Autodesk Inventor part; units mm, degrees
(part 3 of 3)
  point P86 (13.5104, 46.8405)
  point P87 (13.2211, 47.2236)
  point P88 (11.1615, 47.7468)
  point P89 (10.7263, 47.5553)
  point P90 (10.5426, 47.5964)
  point P91 (10.2298, 47.9606)
  point P92 (7.7191, 48.135)
  point P93 (7.5332, 48.1644)
  point P94 (7.1982, 48.5083)
  point P95 (5.0892, 48.7692)
  point P96 (4.6815, 48.5247)
  point P97 (4.4941, 48.5424)
  point P98 (4.1381, 48.8646)
  point P99 (2.0169, 48.9926)
  point P100 (1.6254, 48.7229)
  point P101 (1.4372, 48.7288)
  point P102 (1.0617, 49.028)
  point P103 (-1.0633, 49.0225)
  point P104 (-1.4372, 48.7288)
  point P105 (-1.6254, 48.7229)
  point P106 (-2.0189, 48.9979)
  point P107 (-2.8249, 50.9218)
  point P108 (-4.1394, 48.859)
  point P109 (-4.4941, 48.5424)
  point P110 (-4.6815, 48.5247)
  point P111 (-5.0915, 48.7745)
  point P112 (-6.0168, 50.6439)
  point P113 (-7.5332, 48.1644)
  point P114 (-7.7191, 48.135)
  point P115 (-8.144, 48.3585)
  point P116 (-9.1848, 50.1662)
  point P117 (-10.5426, 47.5964)
  point P118 (-10.7263, 47.5553)
  point P119 (-11.1644, 47.7517)
  point P120 (-12.3167, 49.4905)
  point P121 (-13.5104, 46.8405)
  point P122 (-13.6912, 46.788)
  point P123 (-14.1407, 46.9565)
  point P124 (-15.3999, 48.6194)
  point P125 (-16.1601, 46.2946)
  point P126 (-16.4249, 45.8997)
  point P127 (-16.602, 45.836)
  point P128 (-17.0612, 45.9759)
  point P129 (-18.4224, 47.5565)
  point P130 (-19.2745, 44.7778)
  point P131 (-19.4473, 44.7031)
  point P132 (-19.9144, 44.8139)
  point P133 (-21.3721, 46.3059)
  point P134 (-21.8349, 43.9042)
  point P135 (-22.0481, 43.4792)
  point P136 (-22.2159, 43.3938)
  point P137 (-24.2375, 44.8726)
  point P138 (-24.7347, 42.009)
  point P139 (-24.8967, 41.9132)
  point P140 (-25.3741, 41.9646)
  point P141 (-27.0072, 43.2622)
  point P142 (-27.1654, 40.8213)
  point P143 (-27.3237, 40.373)
  point P144 (-27.4794, 40.2672)
  point P145 (-27.959, 40.2885)
  point P146 (-29.6704, 41.481)
  point P147 (-29.6769, 39.0404)
  point P148 (-29.8048, 38.5777)
  point P149 (-29.9535, 38.4623)
  point P150 (-30.4336, 38.4535)
  point P151 (-32.0674, 37.0947)
  point P152 (-32.1683, 36.6301)
  point P153 (-32.3095, 36.5056)
  point P154 (-32.788, 36.4667)
  point P155 (-34.6354, 37.4352)
  point P156 (-34.4048, 34.5379)
  point P157 (-34.5379, 34.4048)
  point P158 (-35.0131, 34.3359)
  point P159 (-36.9176, 35.1866)
  point P160 (-36.5056, 32.3095)
  point P161 (-36.6301, 32.1683)
  point P162 (-37.1, 32.0697)
  point P163 (-39.0542, 32.7991)
  point P164 (-38.4623, 29.9535)
  point P165 (-38.5777, 29.8048)
  point P166 (-39.0404, 29.6769)
  point P167 (-41.0366, 30.2821)
  point P168 (-40.2851, 27.9545)
  point P169 (-40.2672, 27.4794)
  point P170 (-40.373, 27.3237)
  point P171 (-40.8268, 27.1669)
  point P172 (-42.857, 27.6457)
  point P173 (-41.9132, 24.8967)
  point P174 (-42.009, 24.7347)
  point P175 (-42.4521, 24.5498)
  point P176 (-43.471, 22.685)
  point P177 (-43.3938, 22.2159)
  point P178 (-43.4792, 22.0481)
  point P179 (-43.9098, 21.8358)
  point P180 (-45.984, 22.0563)
  point P181 (-44.7031, 19.4473)
  point P182 (-44.7778, 19.2745)
  point P183 (-45.1942, 19.0356)
  point P184 (-47.2782, 19.1254)
  point P185 (-45.836, 16.602)
  point P186 (-45.8997, 16.4249)
  point P187 (-46.3003, 16.1602)
  point P188 (-48.3858, 16.119)
  point P189 (-46.788, 13.6912)
  point P190 (-46.8405, 13.5104)
  point P191 (-47.2236, 13.2211)
  point P192 (-47.7468, 11.1615)
  point P193 (-47.5553, 10.7263)
  point P194 (-47.5964, 10.5426)
  point P195 (-47.9606, 10.2298)
  point P196 (-50.0245, 9.9276)
  point P197 (-48.135, 7.7191)
  point P198 (-48.1644, 7.5332)
  point P199 (-48.5083, 7.1982)
  constraints: 800 point on circle, 400 centre point, 600 other
extrude "Extrusion1" add sketch "Sketch1" along normal blind 7
sketch "Sketch10" plane through (0, 0, 7) normal (0, 0, 1) x (1, 0, 0)
  arc A0 (8.9575, -3.1642) -> (9.3396, -1.7385) centre (0, 0) ccw
  arc A1 (9.7901, -1.4158) -> (9.3396, -1.7385) centre (9.7328, -1.8117) ccw
  line L0 (9.7901, -1.4158) -> (11.1918, -1.6185)
  spline S0 degree 3 poles (11.1918, -1.6185) (11.2745, -1.6242) (11.5228, -1.6292) (11.9415, -1.5322) knots 0 0 0 0 1 1 1 1
  line L1 (11.1918, -1.6185) -> (11.2745, -1.6242) construction
  line L2 (11.2745, -1.6242) -> (11.5228, -1.6292) construction
  line L3 (11.5228, -1.6292) -> (11.9415, -1.5322) construction
  spline S1 degree 3 poles (11.9415, -1.5322) (12.4367, -1.4162) (13.1438, -1.1571) (13.9903, -0.5909) knots 0 0 0 0 1 1 1 1
  line L4 (11.9415, -1.5322) -> (12.4367, -1.4162) construction
  line L5 (12.4367, -1.4162) -> (13.1438, -1.1571) construction
  line L6 (13.1438, -1.1571) -> (13.9903, -0.5909) construction
  arc A2 (13.9903, -0.5909) -> (13.9903, 0.5909) centre (0, 0) ccw
  spline S2 degree 3 poles (13.9903, 0.5909) (13.1438, 1.1571) (12.4367, 1.4162) (11.9415, 1.5322) knots 0 0 0 0 1 1 1 1
  line L7 (13.9903, 0.5909) -> (13.1438, 1.1571) construction
  line L8 (13.1438, 1.1571) -> (12.4367, 1.4162) construction
  line L9 (12.4367, 1.4162) -> (11.9415, 1.5322) construction
  spline S3 degree 3 poles (11.9415, 1.5322) (11.5228, 1.6292) (11.2745, 1.6242) (11.1918, 1.6185) knots 0 0 0 0 1 1 1 1
  line L10 (11.9415, 1.5322) -> (11.5228, 1.6292) construction
  line L11 (11.5228, 1.6292) -> (11.2745, 1.6242) construction
  line L12 (11.2745, 1.6242) -> (11.1918, 1.6185) construction
  line L13 (11.1918, 1.6185) -> (9.7901, 1.4158)
  arc A3 (9.3396, 1.7385) -> (9.7901, 1.4158) centre (9.7328, 1.8117) ccw
  arc A4 (9.3396, 1.7385) -> (8.9575, 3.1642) centre (0, 0) ccw
  arc A5 (9.1863, 3.6689) -> (8.9575, 3.1642) centre (9.3347, 3.2975) ccw
  line L14 (9.1863, 3.6689) -> (10.5016, 4.1942)
  spline S4 degree 3 poles (10.5016, 4.1942) (10.5761, 4.2307) (10.7937, 4.3505) (11.1078, 4.6438) knots 0 0 0 0 1 1 1 1
  line L15 (10.5016, 4.1942) -> (10.5761, 4.2307) construction
  line L16 (10.5761, 4.2307) -> (10.7937, 4.3505) construction
  line L17 (10.7937, 4.3505) -> (11.1078, 4.6438) construction
  spline S5 degree 3 poles (11.1078, 4.6438) (11.4787, 4.9919) (11.9614, 5.5698) (12.4114, 6.4834) knots 0 0 0 0 1 1 1 1
  line L18 (11.1078, 4.6438) -> (11.4787, 4.9919) construction
  line L19 (11.4787, 4.9919) -> (11.9614, 5.5698) construction
  line L20 (11.9614, 5.5698) -> (12.4114, 6.4834) construction
  arc A6 (12.4114, 6.4834) -> (11.8204, 7.5069) centre (0, 0) ccw
  spline S6 degree 3 poles (11.8204, 7.5069) (10.8043, 7.5739) (10.0624, 7.4449) (9.5755, 7.2977) knots 0 0 0 0 1 1 1 1
  line L21 (11.8204, 7.5069) -> (10.8043, 7.5739) construction
  line L22 (10.8043, 7.5739) -> (10.0624, 7.4449) construction
  line L23 (10.0624, 7.4449) -> (9.5755, 7.2977) construction
  spline S7 degree 3 poles (9.5755, 7.2977) (9.1645, 7.1723) (8.9519, 7.0438) (8.8831, 6.9975) knots 0 0 0 0 1 1 1 1
  line L24 (9.5755, 7.2977) -> (9.1645, 7.1723) construction
  line L25 (9.1645, 7.1723) -> (8.9519, 7.0438) construction
  line L26 (8.9519, 7.0438) -> (8.8831, 6.9975) construction
  line L27 (8.8831, 6.9975) -> (7.7706, 6.1211)
  arc A7 (7.2191, 6.1753) -> (7.7706, 6.1211) centre (7.523, 6.4354) ccw
  arc A8 (7.2191, 6.1753) -> (6.1753, 7.2191) centre (0, 0) ccw
  arc A9 (6.1211, 7.7706) -> (6.1753, 7.2191) centre (6.4354, 7.523) ccw
  line L28 (6.1211, 7.7706) -> (6.9975, 8.8831)
  spline S8 degree 3 poles (6.9975, 8.8831) (7.0438, 8.9519) (7.1723, 9.1645) (7.2977, 9.5755) knots 0 0 0 0 1 1 1 1
  line L29 (6.9975, 8.8831) -> (7.0438, 8.9519) construction
  line L30 (7.0438, 8.9519) -> (7.1723, 9.1645) construction
  line L31 (7.1723, 9.1645) -> (7.2977, 9.5755) construction
  spline S9 degree 3 poles (7.2977, 9.5755) (7.4449, 10.0624) (7.5739, 10.8043) (7.5069, 11.8204) knots 0 0 0 0 1 1 1 1
  line L32 (7.2977, 9.5755) -> (7.4449, 10.0624) construction
  line L33 (7.4449, 10.0624) -> (7.5739, 10.8043) construction
  line L34 (7.5739, 10.8043) -> (7.5069, 11.8204) construction
  arc A10 (7.5069, 11.8204) -> (6.4834, 12.4114) centre (0, 0) ccw
  spline S10 degree 3 poles (6.4834, 12.4114) (5.5698, 11.9614) (4.9919, 11.4787) (4.6438, 11.1078) knots 0 0 0 0 1 1 1 1
  line L35 (6.4834, 12.4114) -> (5.5698, 11.9614) construction
  line L36 (5.5698, 11.9614) -> (4.9919, 11.4787) construction
  line L37 (4.9919, 11.4787) -> (4.6438, 11.1078) construction
  spline S11 degree 3 poles (4.6438, 11.1078) (4.3505, 10.7937) (4.2307, 10.5761) (4.1942, 10.5016) knots 0 0 0 0 1 1 1 1
  line L38 (4.6438, 11.1078) -> (4.3505, 10.7937) construction
  line L39 (4.3505, 10.7937) -> (4.2307, 10.5761) construction
  line L40 (4.2307, 10.5761) -> (4.1942, 10.5016) construction
  line L41 (4.1942, 10.5016) -> (3.6689, 9.1863)
  arc A11 (3.1642, 8.9575) -> (3.6689, 9.1863) centre (3.2975, 9.3347) ccw
  arc A12 (3.1642, 8.9575) -> (1.7385, 9.3396) centre (0, 0) ccw
  arc A13 (1.4158, 9.7901) -> (1.7385, 9.3396) centre (1.8117, 9.7328) ccw
  line L42 (1.4158, 9.7901) -> (1.6185, 11.1918)
  spline S12 degree 3 poles (1.6185, 11.1918) (1.6242, 11.2745) (1.6292, 11.5228) (1.5322, 11.9415) knots 0 0 0 0 1 1 1 1
  line L43 (1.6185, 11.1918) -> (1.6242, 11.2745) construction
  line L44 (1.6242, 11.2745) -> (1.6292, 11.5228) construction
  line L45 (1.6292, 11.5228) -> (1.5322, 11.9415) construction
  spline S13 degree 3 poles (1.5322, 11.9415) (1.4162, 12.4367) (1.1571, 13.1438) (0.5909, 13.9903) knots 0 0 0 0 1 1 1 1
  line L46 (1.5322, 11.9415) -> (1.4162, 12.4367) construction
  line L47 (1.4162, 12.4367) -> (1.1571, 13.1438) construction
  line L48 (1.1571, 13.1438) -> (0.5909, 13.9903) construction
  arc A14 (0.5909, 13.9903) -> (-0.5909, 13.9903) centre (0, 0) ccw
  spline S14 degree 3 poles (-0.5909, 13.9903) (-1.1571, 13.1438) (-1.4162, 12.4367) (-1.5322, 11.9415) knots 0 0 0 0 1 1 1 1
  line L49 (-0.5909, 13.9903) -> (-1.1571, 13.1438) construction
  line L50 (-1.1571, 13.1438) -> (-1.4162, 12.4367) construction
  line L51 (-1.4162, 12.4367) -> (-1.5322, 11.9415) construction
  spline S15 degree 3 poles (-1.5322, 11.9415) (-1.6292, 11.5228) (-1.6242, 11.2745) (-1.6185, 11.1918) knots 0 0 0 0 1 1 1 1
  line L52 (-1.5322, 11.9415) -> (-1.6292, 11.5228) construction
  line L53 (-1.6292, 11.5228) -> (-1.6242, 11.2745) construction
  line L54 (-1.6242, 11.2745) -> (-1.6185, 11.1918) construction
  line L55 (-1.6185, 11.1918) -> (-1.4158, 9.7901)
  arc A15 (-1.7385, 9.3396) -> (-1.4158, 9.7901) centre (-1.8117, 9.7328) ccw
  arc A16 (-1.7385, 9.3396) -> (-3.1642, 8.9575) centre (0, 0) ccw
  arc A17 (-3.6689, 9.1863) -> (-3.1642, 8.9575) centre (-3.2975, 9.3347) ccw
  line L56 (-3.6689, 9.1863) -> (-4.1942, 10.5016)
  spline S16 degree 3 poles (-4.1942, 10.5016) (-4.2307, 10.5761) (-4.3505, 10.7937) (-4.6438, 11.1078) knots 0 0 0 0 1 1 1 1
  line L57 (-4.1942, 10.5016) -> (-4.2307, 10.5761) construction
  line L58 (-4.2307, 10.5761) -> (-4.3505, 10.7937) construction
  line L59 (-4.3505, 10.7937) -> (-4.6438, 11.1078) construction
  spline S17 degree 3 poles (-4.6438, 11.1078) (-4.9919, 11.4787) (-5.5698, 11.9614) (-6.4834, 12.4114) knots 0 0 0 0 1 1 1 1
  line L60 (-4.6438, 11.1078) -> (-4.9919, 11.4787) construction
  line L61 (-4.9919, 11.4787) -> (-5.5698, 11.9614) construction
  line L62 (-5.5698, 11.9614) -> (-6.4834, 12.4114) construction
  arc A18 (-6.4834, 12.4114) -> (-7.5069, 11.8204) centre (0, 0) ccw
  spline S18 degree 3 poles (-7.5069, 11.8204) (-7.5739, 10.8043) (-7.4449, 10.0624) (-7.2977, 9.5755) knots 0 0 0 0 1 1 1 1
  line L63 (-7.5069, 11.8204) -> (-7.5739, 10.8043) construction
  line L64 (-7.5739, 10.8043) -> (-7.4449, 10.0624) construction
  line L65 (-7.4449, 10.0624) -> (-7.2977, 9.5755) construction
  spline S19 degree 3 poles (-7.2977, 9.5755) (-7.1723, 9.1645) (-7.0438, 8.9519) (-6.9975, 8.8831) knots 0 0 0 0 1 1 1 1
  line L66 (-7.2977, 9.5755) -> (-7.1723, 9.1645) construction
  line L67 (-7.1723, 9.1645) -> (-7.0438, 8.9519) construction
  line L68 (-7.0438, 8.9519) -> (-6.9975, 8.8831) construction
  line L69 (-6.9975, 8.8831) -> (-6.1211, 7.7706)
  arc A19 (-6.1753, 7.2191) -> (-6.1211, 7.7706) centre (-6.4354, 7.523) ccw
  arc A20 (-6.1753, 7.2191) -> (-7.2191, 6.1753) centre (0, 0) ccw
  arc A21 (-7.7706, 6.1211) -> (-7.2191, 6.1753) centre (-7.523, 6.4354) ccw
  line L70 (-7.7706, 6.1211) -> (-8.8831, 6.9975)
  spline S20 degree 3 poles (-8.8831, 6.9975) (-8.9519, 7.0438) (-9.1645, 7.1723) (-9.5755, 7.2977) knots 0 0 0 0 1 1 1 1
  line L71 (-8.8831, 6.9975) -> (-8.9519, 7.0438) construction
  line L72 (-8.9519, 7.0438) -> (-9.1645, 7.1723) construction
  line L73 (-9.1645, 7.1723) -> (-9.5755, 7.2977) construction
  spline S21 degree 3 poles (-9.5755, 7.2977) (-10.0624, 7.4449) (-10.8043, 7.5739) (-11.8204, 7.5069) knots 0 0 0 0 1 1 1 1
  line L74 (-9.5755, 7.2977) -> (-10.0624, 7.4449) construction
  line L75 (-10.0624, 7.4449) -> (-10.8043, 7.5739) construction
  line L76 (-10.8043, 7.5739) -> (-11.8204, 7.5069) construction
  arc A22 (-11.8204, 7.5069) -> (-12.4114, 6.4834) centre (0, 0) ccw
  spline S22 degree 3 poles (-12.4114, 6.4834) (-11.9614, 5.5698) (-11.4787, 4.9919) (-11.1078, 4.6438) knots 0 0 0 0 1 1 1 1
  line L77 (-12.4114, 6.4834) -> (-11.9614, 5.5698) construction
  line L78 (-11.9614, 5.5698) -> (-11.4787, 4.9919) construction
  line L79 (-11.4787, 4.9919) -> (-11.1078, 4.6438) construction
  spline S23 degree 3 poles (-11.1078, 4.6438) (-10.7937, 4.3505) (-10.5761, 4.2307) (-10.5016, 4.1942) knots 0 0 0 0 1 1 1 1
  line L80 (-11.1078, 4.6438) -> (-10.7937, 4.3505) construction
  line L81 (-10.7937, 4.3505) -> (-10.5761, 4.2307) construction
  line L82 (-10.5761, 4.2307) -> (-10.5016, 4.1942) construction
  line L83 (-10.5016, 4.1942) -> (-9.1863, 3.6689)
  arc A23 (-8.9575, 3.1642) -> (-9.1863, 3.6689) centre (-9.3347, 3.2975) ccw
  arc A24 (-8.9575, 3.1642) -> (-9.3396, 1.7385) centre (0, 0) ccw
  arc A25 (-9.7901, 1.4158) -> (-9.3396, 1.7385) centre (-9.7328, 1.8117) ccw
  line L84 (-9.7901, 1.4158) -> (-11.1918, 1.6185)
  spline S24 degree 3 poles (-11.1918, 1.6185) (-11.2745, 1.6242) (-11.5228, 1.6292) (-11.9415, 1.5322) knots 0 0 0 0 1 1 1 1
  line L85 (-11.1918, 1.6185) -> (-11.2745, 1.6242) construction
  line L86 (-11.2745, 1.6242) -> (-11.5228, 1.6292) construction
  line L87 (-11.5228, 1.6292) -> (-11.9415, 1.5322) construction
  spline S25 degree 3 poles (-11.9415, 1.5322) (-12.4367, 1.4162) (-13.1438, 1.1571) (-13.9903, 0.5909) knots 0 0 0 0 1 1 1 1
  line L88 (-11.9415, 1.5322) -> (-12.4367, 1.4162) construction
  line L89 (-12.4367, 1.4162) -> (-13.1438, 1.1571) construction
  line L90 (-13.1438, 1.1571) -> (-13.9903, 0.5909) construction
  arc A26 (-13.9903, 0.5909) -> (-13.9903, -0.5909) centre (0, 0) ccw
  spline S26 degree 3 poles (-13.9903, -0.5909) (-13.1438, -1.1571) (-12.4367, -1.4162) (-11.9415, -1.5322) knots 0 0 0 0 1 1 1 1
  line L91 (-13.9903, -0.5909) -> (-13.1438, -1.1571) construction
  line L92 (-13.1438, -1.1571) -> (-12.4367, -1.4162) construction
  line L93 (-12.4367, -1.4162) -> (-11.9415, -1.5322) construction
  spline S27 degree 3 poles (-11.9415, -1.5322) (-11.5228, -1.6292) (-11.2745, -1.6242) (-11.1918, -1.6185) knots 0 0 0 0 1 1 1 1
  line L94 (-11.9415, -1.5322) -> (-11.5228, -1.6292) construction
  line L95 (-11.5228, -1.6292) -> (-11.2745, -1.6242) construction
  line L96 (-11.2745, -1.6242) -> (-11.1918, -1.6185) construction
  line L97 (-11.1918, -1.6185) -> (-9.7901, -1.4158)
  arc A27 (-9.3396, -1.7385) -> (-9.7901, -1.4158) centre (-9.7328, -1.8117) ccw
  arc A28 (-9.3396, -1.7385) -> (-8.9575, -3.1642) centre (0, 0) ccw
  arc A29 (-9.1863, -3.6689) -> (-8.9575, -3.1642) centre (-9.3347, -3.2975) ccw
  line L98 (-9.1863, -3.6689) -> (-10.5016, -4.1942)
  spline S28 degree 3 poles (-10.5016, -4.1942) (-10.5761, -4.2307) (-10.7937, -4.3505) (-11.1078, -4.6438) knots 0 0 0 0 1 1 1 1
  line L99 (-10.5016, -4.1942) -> (-10.5761, -4.2307) construction
  line L100 (-10.5761, -4.2307) -> (-10.7937, -4.3505) construction
  line L101 (-10.7937, -4.3505) -> (-11.1078, -4.6438) construction
  spline S29 degree 3 poles (-11.1078, -4.6438) (-11.4787, -4.9919) (-11.9614, -5.5698) (-12.4114, -6.4834) knots 0 0 0 0 1 1 1 1
  line L102 (-11.1078, -4.6438) -> (-11.4787, -4.9919) construction
  line L103 (-11.4787, -4.9919) -> (-11.9614, -5.5698) construction
  line L104 (-11.9614, -5.5698) -> (-12.4114, -6.4834) construction
  arc A30 (-12.4114, -6.4834) -> (-11.8204, -7.5069) centre (0, 0) ccw
  spline S30 degree 3 poles (-11.8204, -7.5069) (-10.8043, -7.5739) (-10.0624, -7.4449) (-9.5755, -7.2977) knots 0 0 0 0 1 1 1 1
  line L105 (-11.8204, -7.5069) -> (-10.8043, -7.5739) construction
  line L106 (-10.8043, -7.5739) -> (-10.0624, -7.4449) construction
  line L107 (-10.0624, -7.4449) -> (-9.5755, -7.2977) construction
  spline S31 degree 3 poles (-9.5755, -7.2977) (-9.1645, -7.1723) (-8.9519, -7.0438) (-8.8831, -6.9975) knots 0 0 0 0 1 1 1 1
  line L108 (-9.5755, -7.2977) -> (-9.1645, -7.1723) construction
  line L109 (-9.1645, -7.1723) -> (-8.9519, -7.0438) construction
  line L110 (-8.9519, -7.0438) -> (-8.8831, -6.9975) construction
  line L111 (-8.8831, -6.9975) -> (-7.7706, -6.1211)
  arc A31 (-7.2191, -6.1753) -> (-7.7706, -6.1211) centre (-7.523, -6.4354) ccw
  arc A32 (-7.2191, -6.1753) -> (-6.1753, -7.2191) centre (0, 0) ccw
  arc A33 (-6.1211, -7.7706) -> (-6.1753, -7.2191) centre (-6.4354, -7.523) ccw
  line L112 (-6.1211, -7.7706) -> (-6.9975, -8.8831)
  spline S32 degree 3 poles (-6.9975, -8.8831) (-7.0438, -8.9519) (-7.1723, -9.1645) (-7.2977, -9.5755) knots 0 0 0 0 1 1 1 1
  line L113 (-6.9975, -8.8831) -> (-7.0438, -8.9519) construction
  line L114 (-7.0438, -8.9519) -> (-7.1723, -9.1645) construction
  line L115 (-7.1723, -9.1645) -> (-7.2977, -9.5755) construction
  spline S33 degree 3 poles (-7.2977, -9.5755) (-7.4449, -10.0624) (-7.5739, -10.8043) (-7.5069, -11.8204) knots 0 0 0 0 1 1 1 1
  line L116 (-7.2977, -9.5755) -> (-7.4449, -10.0624) construction
  line L117 (-7.4449, -10.0624) -> (-7.5739, -10.8043) construction
  line L118 (-7.5739, -10.8043) -> (-7.5069, -11.8204) construction
  arc A34 (-7.5069, -11.8204) -> (-6.4834, -12.4114) centre (0, 0) ccw
  spline S34 degree 3 poles (-6.4834, -12.4114) (-5.5698, -11.9614) (-4.9919, -11.4787) (-4.6438, -11.1078) knots 0 0 0 0 1 1 1 1
  line L119 (-6.4834, -12.4114) -> (-5.5698, -11.9614) construction
  line L120 (-5.5698, -11.9614) -> (-4.9919, -11.4787) construction
  line L121 (-4.9919, -11.4787) -> (-4.6438, -11.1078) construction
  spline S35 degree 3 poles (-4.6438, -11.1078) (-4.3505, -10.7937) (-4.2307, -10.5761) (-4.1942, -10.5016) knots 0 0 0 0 1 1 1 1
  line L122 (-4.6438, -11.1078) -> (-4.3505, -10.7937) construction
  line L123 (-4.3505, -10.7937) -> (-4.2307, -10.5761) construction
  line L124 (-4.2307, -10.5761) -> (-4.1942, -10.5016) construction
  line L125 (-4.1942, -10.5016) -> (-3.6689, -9.1863)
  arc A35 (-3.1642, -8.9575) -> (-3.6689, -9.1863) centre (-3.2975, -9.3347) ccw
  arc A36 (-3.1642, -8.9575) -> (-1.7385, -9.3396) centre (0, 0) ccw
  arc A37 (-1.4158, -9.7901) -> (-1.7385, -9.3396) centre (-1.8117, -9.7328) ccw
  line L126 (-1.4158, -9.7901) -> (-1.6185, -11.1918)
  spline S36 degree 3 poles (-1.6185, -11.1918) (-1.6242, -11.2745) (-1.6292, -11.5228) (-1.5322, -11.9415) knots 0 0 0 0 1 1 1 1
  line L127 (-1.6185, -11.1918) -> (-1.6242, -11.2745) construction
  line L128 (-1.6242, -11.2745) -> (-1.6292, -11.5228) construction
  line L129 (-1.6292, -11.5228) -> (-1.5322, -11.9415) construction
  spline S37 degree 3 poles (-1.5322, -11.9415) (-1.4162, -12.4367) (-1.1571, -13.1438) (-0.5909, -13.9903) knots 0 0 0 0 1 1 1 1
  line L130 (-1.5322, -11.9415) -> (-1.4162, -12.4367) construction
  line L131 (-1.4162, -12.4367) -> (-1.1571, -13.1438) construction
  line L132 (-1.1571, -13.1438) -> (-0.5909, -13.9903) construction
  arc A38 (-0.5909, -13.9903) -> (0.5909, -13.9903) centre (0, 0) ccw
  spline S38 degree 3 poles (0.5909, -13.9903) (1.1571, -13.1438) (1.4162, -12.4367) (1.5322, -11.9415) knots 0 0 0 0 1 1 1 1
  line L133 (0.5909, -13.9903) -> (1.1571, -13.1438) construction
  line L134 (1.1571, -13.1438) -> (1.4162, -12.4367) construction
  line L135 (1.4162, -12.4367) -> (1.5322, -11.9415) construction
  spline S39 degree 3 poles (1.5322, -11.9415) (1.6292, -11.5228) (1.6242, -11.2745) (1.6185, -11.1918) knots 0 0 0 0 1 1 1 1
  line L136 (1.5322, -11.9415) -> (1.6292, -11.5228) construction
  line L137 (1.6292, -11.5228) -> (1.6242, -11.2745) construction
  line L138 (1.6242, -11.2745) -> (1.6185, -11.1918) construction
  line L139 (1.6185, -11.1918) -> (1.4158, -9.7901)
  arc A39 (1.7385, -9.3396) -> (1.4158, -9.7901) centre (1.8117, -9.7328) ccw
  arc A40 (1.7385, -9.3396) -> (3.1642, -8.9575) centre (0, 0) ccw
  arc A41 (3.6689, -9.1863) -> (3.1642, -8.9575) centre (3.2975, -9.3347) ccw
  line L140 (3.6689, -9.1863) -> (4.1942, -10.5016)
  spline S40 degree 3 poles (4.1942, -10.5016) (4.2307, -10.5761) (4.3505, -10.7937) (4.6438, -11.1078) knots 0 0 0 0 1 1 1 1
  line L141 (4.1942, -10.5016) -> (4.2307, -10.5761) construction
  line L142 (4.2307, -10.5761) -> (4.3505, -10.7937) construction
  line L143 (4.3505, -10.7937) -> (4.6438, -11.1078) construction
  spline S41 degree 3 poles (4.6438, -11.1078) (4.9919, -11.4787) (5.5698, -11.9614) (6.4834, -12.4114) knots 0 0 0 0 1 1 1 1
  line L144 (4.6438, -11.1078) -> (4.9919, -11.4787) construction
  line L145 (4.9919, -11.4787) -> (5.5698, -11.9614) construction
  line L146 (5.5698, -11.9614) -> (6.4834, -12.4114) construction
  arc A42 (6.4834, -12.4114) -> (7.5069, -11.8204) centre (0, 0) ccw
  spline S42 degree 3 poles (7.5069, -11.8204) (7.5739, -10.8043) (7.4449, -10.0624) (7.2977, -9.5755) knots 0 0 0 0 1 1 1 1
  line L147 (7.5069, -11.8204) -> (7.5739, -10.8043) construction
  line L148 (7.5739, -10.8043) -> (7.4449, -10.0624) construction
  line L149 (7.4449, -10.0624) -> (7.2977, -9.5755) construction
  spline S43 degree 3 poles (7.2977, -9.5755) (7.1723, -9.1645) (7.0438, -8.9519) (6.9975, -8.8831) knots 0 0 0 0 1 1 1 1
  line L150 (7.2977, -9.5755) -> (7.1723, -9.1645) construction
  line L151 (7.1723, -9.1645) -> (7.0438, -8.9519) construction
  line L152 (7.0438, -8.9519) -> (6.9975, -8.8831) construction
  line L153 (6.9975, -8.8831) -> (6.1211, -7.7706)
  arc A43 (6.1753, -7.2191) -> (6.1211, -7.7706) centre (6.4354, -7.523) ccw
  arc A44 (6.1753, -7.2191) -> (7.2191, -6.1753) centre (0, 0) ccw
  arc A45 (7.7706, -6.1211) -> (7.2191, -6.1753) centre (7.523, -6.4354) ccw
  line L154 (7.7706, -6.1211) -> (8.8831, -6.9975)
  spline S44 degree 3 poles (8.8831, -6.9975) (8.9519, -7.0438) (9.1645, -7.1723) (9.5755, -7.2977) knots 0 0 0 0 1 1 1 1
  line L155 (8.8831, -6.9975) -> (8.9519, -7.0438) construction
  line L156 (8.9519, -7.0438) -> (9.1645, -7.1723) construction
  line L157 (9.1645, -7.1723) -> (9.5755, -7.2977) construction
  spline S45 degree 3 poles (9.5755, -7.2977) (10.0624, -7.4449) (10.8043, -7.5739) (11.8204, -7.5069) knots 0 0 0 0 1 1 1 1
  line L158 (9.5755, -7.2977) -> (10.0624, -7.4449) construction
  line L159 (10.0624, -7.4449) -> (10.8043, -7.5739) construction
  line L160 (10.8043, -7.5739) -> (11.8204, -7.5069) construction
  arc A46 (11.8204, -7.5069) -> (12.4114, -6.4834) centre (0, 0) ccw
  spline S46 degree 3 poles (12.4114, -6.4834) (11.9614, -5.5698) (11.4787, -4.9919) (11.1078, -4.6438) knots 0 0 0 0 1 1 1 1
  line L161 (12.4114, -6.4834) -> (11.9614, -5.5698) construction
  line L162 (11.9614, -5.5698) -> (11.4787, -4.9919) construction
  line L163 (11.4787, -4.9919) -> (11.1078, -4.6438) construction
  spline S47 degree 3 poles (11.1078, -4.6438) (10.7937, -4.3505) (10.5761, -4.2307) (10.5016, -4.1942) knots 0 0 0 0 1 1 1 1
  line L164 (11.1078, -4.6438) -> (10.7937, -4.3505) construction
  line L165 (10.7937, -4.3505) -> (10.5761, -4.2307) construction
  line L166 (10.5761, -4.2307) -> (10.5016, -4.1942) construction
  line L167 (10.5016, -4.1942) -> (9.1863, -3.6689)
  arc A47 (8.9575, -3.1642) -> (9.1863, -3.6689) centre (9.3347, -3.2975) ccw
  point P0 (7.7706, -6.1211)
  point P1 (8.8898, -7.002)
  point P2 (9.5813, -7.2995)
  point P3 (11.8204, -7.5069)
  point P4 (11.1078, -4.6438)
  point P5 (9.1863, -3.6689)
  point P6 (8.9575, -3.1642)
  point P7 (9.3396, -1.7385)
  point P8 (9.7901, -1.4158)
  point P9 (11.1997, -1.619)
  point P10 (11.9474, -1.5308)
  point P11 (11.9415, 1.5322)
  point P12 (11.1918, 1.6185)
  point P13 (9.7901, 1.4158)
  point P14 (9.3396, 1.7385)
  point P15 (8.9575, 3.1642)
  point P16 (9.1863, 3.6689)
  point P17 (10.5088, 4.1978)
  point P18 (11.1122, 4.648)
  point P19 (9.5755, 7.2977)
  point P20 (8.8831, 6.9975)
  point P21 (7.7706, 6.1211)
  point P22 (7.2191, 6.1753)
  point P23 (6.1753, 7.2191)
  point P24 (6.1211, 7.7706)
  point P25 (7.002, 8.8898)
  point P26 (7.2995, 9.5813)
  point P27 (4.6438, 11.1078)
  point P28 (3.6689, 9.1863)
  point P29 (3.1642, 8.9575)
  point P30 (1.7385, 9.3396)
  point P31 (1.4158, 9.7901)
  point P32 (1.619, 11.1997)
  point P33 (1.5308, 11.9474)
  point P34 (-1.5322, 11.9415)
  point P35 (-1.6185, 11.1918)
  point P36 (-1.4158, 9.7901)
  point P37 (-1.7385, 9.3396)
  point P38 (-3.1642, 8.9575)
  point P39 (-3.6689, 9.1863)
  point P40 (-4.1978, 10.5088)
  point P41 (-4.648, 11.1122)
  point P42 (-6.4834, 12.4114)
  point P43 (-7.2977, 9.5755)
  point P44 (-6.9975, 8.8831)
  point P45 (-6.1211, 7.7706)
  point P46 (-6.1753, 7.2191)
  point P47 (-7.2191, 6.1753)
  point P48 (-7.7706, 6.1211)
  point P49 (-8.8898, 7.002)
  point P50 (-9.5813, 7.2995)
  point P51 (-11.8204, 7.5069)
  point P52 (-11.1078, 4.6438)
  point P53 (-9.1863, 3.6689)
  point P54 (-8.9575, 3.1642)
  point P55 (-9.3396, 1.7385)
  point P56 (-9.7901, 1.4158)
  point P57 (-11.1997, 1.619)
  point P58 (-11.9474, 1.5308)
  point P59 (-11.9415, -1.5322)
  point P60 (-11.1918, -1.6185)
  point P61 (-9.7901, -1.4158)
  point P62 (-9.3396, -1.7385)
  point P63 (-8.9575, -3.1642)
  point P64 (-9.1863, -3.6689)
  point P65 (-10.5088, -4.1978)
  point P66 (-11.1122, -4.648)
  point P67 (-12.4114, -6.4834)
  point P68 (-9.5755, -7.2977)
  point P69 (-8.8831, -6.9975)
  point P70 (-7.7706, -6.1211)
  point P71 (-7.2191, -6.1753)
  point P72 (-6.1753, -7.2191)
  point P73 (-6.1211, -7.7706)
  point P74 (-7.002, -8.8898)
  point P75 (-7.2995, -9.5813)
  point P76 (-7.5069, -11.8204)
  point P77 (-4.6438, -11.1078)
  point P78 (-3.6689, -9.1863)
  point P79 (-3.1642, -8.9575)
  point P80 (-1.7385, -9.3396)
  point P81 (-1.4158, -9.7901)
  point P82 (-1.619, -11.1997)
  point P83 (-1.5308, -11.9474)
  point P84 (1.5308, -11.9474)
  point P85 (1.6185, -11.1918)
  point P86 (1.4158, -9.7901)
  point P87 (1.7385, -9.3396)
  point P88 (3.1642, -8.9575)
  point P89 (3.6689, -9.1863)
  point P90 (4.1978, -10.5088)
  point P91 (4.648, -11.1122)
  point P92 (7.2977, -9.5755)
  point P93 (6.9975, -8.8831)
  point P94 (6.1211, -7.7706)
  point P95 (6.1753, -7.2191)
  point P96 (7.2191, -6.1753)
  constraints: 96 point on circle, 48 centre point, 48 end point, 144 other
extrude "Extrusion10" add sketch "Sketch10" along normal blind 8
sketch "Sketch11" plane through (0, 0, 15) normal (0, 0, 1) x (1, 0, 0)
  circle A0 centre (0, 0) radius 4
  dimension "d24" = 8
  constraints: 1 centre point, 1 coincident
  measures "d24" diameter of A0
extrude "Extrusion11" cut sketch "Sketch11" against normal blind 20
body "Solid1"
